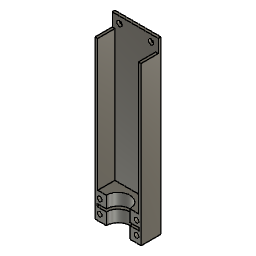
platform_bottom (Autodesk Fusion 360 design; units mm, degrees)
Autodesk Fusion 360 part; units mm, degrees
sketch "スケッチ1" plane through (0, 0, 0) normal (0, 0, 1) x (1, 0, 0)
  line L0 (-17.5, 15) -> (17.5, 15)
  line L1 (17.5, 15) -> (17.5, 0)
  line L2 (17.5, 0) -> (-17.5, 0)
  line L3 (-17.5, 0) -> (-17.5, 15)
  dimension "d1" = 35
  dimension "d2" = 15
  constraint horizontal L0
  constraint vertical L1
  constraint horizontal L2
  constraint vertical L3
  constraint midpoint origin L2
  measures "d1" distance of L0.start L0.end
  measures "d2" distance of L0.start L2.end
extrude "押し出し1" add sketch "スケッチ1" along normal blind 120
sketch "スケッチ2" plane through (0, 0, 0) normal (0, 0, -1) x (1, 0, 0)
  line L0 (17.5, 0) -> (-17.5, 0)
  line L1 (-17.5, 0) -> (-17.5, -15)
  line L2 (-17.5, -15) -> (17.5, -15)
  line L3 (17.5, -15) -> (17.5, 0)
  circle A0 centre (0, 0) radius 9
  dimension "d5" = 18
  constraint coincident A0.centre origin
  measures "d5" diameter of A0
extrude "押し出し2" cut sketch "スケッチ2" against normal blind 20 contours L0 A0 picked at (1.5, -2.5981)
sketch "スケッチ3" plane through (0, 0, 120) normal (0, 0, 1) x (-1, 0, 0)
  line L0 (17.5, 0) -> (-17.5, 0)
  line L1 (-17.5, 0) -> (-17.5, -15)
  line L2 (-17.5, -15) -> (17.5, -15)
  line L3 (17.5, -15) -> (17.5, 0)
  line L4 (15.5, -13) -> (-15.5, -13)
  line L5 (-15.5, -13) -> (-15.5, 0)
  line L6 (-15.5, 0) -> (15.5, 0)
  line L7 (15.5, 0) -> (15.5, -13)
  dimension "d8" = 2
  dimension "d9" = 31
  constraint horizontal L4
  constraint vertical L5
  constraint horizontal L6
  constraint vertical L7
  constraint coincident L0 L5.end
  constraint midpoint origin L6
  measures "d8" distance of L2 L4
  measures "d9" distance of L5 L7
extrude "押し出し3" cut sketch "スケッチ3" against normal blind 100 contours L0 L4 L5 L6 L7
ref_plane "作業平面1" through (0, 7.5, 9) normal (0, 0, -1) x (-1, 0, 0)
sketch "スケッチ4" plane through (0, 6, 9) normal (0, 0, -1) x (1, 0, 0)
  line L0 (-17.5, 6) -> (17.5, 6)
  line L1 (17.5, 6) -> (17.5, -5)
  line L2 (17.5, -5) -> (-17.5, -5)
  line L3 (-17.5, -5) -> (-17.5, 6)
  line L4 (-17.5, 6) -> (-17.5, -9)
  line L5 (17.5, -9) -> (17.5, 6)
  line L6 (17.5, 6) -> (9, 6)
  dimension "d13" = 11
  constraint horizontal L0
  constraint vertical L1
  constraint horizontal L2
  constraint vertical L3
  constraint collinear L3 L4
  constraint collinear L1 L5
  constraint collinear L0 L6
  measures "d13" distance of L0 L2
extrude "押し出し4" cut sketch "スケッチ4" against normal blind 2
sketch "スケッチ5" plane through (0, 15, 0) normal (0, 1, 0) x (-1, 0, 0)
  line L0 (-17.5, 0) -> (17.5, 0)
  line L1 (17.5, 0) -> (17.5, 120)
  line L2 (17.5, 120) -> (-17.5, 120)
  line L3 (-17.5, 120) -> (-17.5, 0)
  line L4 (-17.5, 130) -> (17.5, 130)
  line L5 (17.5, 130) -> (17.5, 120)
  line L6 (17.5, 120) -> (-17.5, 120)
  line L7 (-17.5, 120) -> (-17.5, 130)
  line L8 (-17.5, 125) -> (17.5, 125) construction
  circle A0 centre (12, 125) radius 2
  circle A1 centre (-12, 125) radius 2
  dimension "d16" = 4
  dimension "d17" = 4
  dimension "d18" = 24
  dimension "d19" = 10
  dimension "d20" = 5.5
  constraint horizontal L4
  constraint vertical L5
  constraint horizontal L6
  constraint vertical L7
  constraint collinear L2 L6
  constraint midpoint L7 L8.start
  constraint midpoint L5 L8.end
  constraint coincident L8 A0.centre
  constraint coincident L8 A1.centre
  constraint collinear L3 L7
  constraint collinear L1 L5
  measures "d16" diameter of A1
  measures "d17" diameter of A0
  measures "d18" distance of A0.centre A1.centre
  measures "d19" distance of L4.start L2.end
  measures "d20" distance of L8.end A0.centre
extrude "押し出し5" add sketch "スケッチ5" against normal blind 2 contours L2 L4 L5 L6 L7
sketch "スケッチ7" plane through (0, 0, 0) normal (0, -1, 0) x (1, 0, 0)
  line L0 (-17.5, 11) -> (-9, 11)
  line L1 (-9, 11) -> (-9, 20)
  line L2 (-9, 20) -> (-15.5, 20)
  line L3 (-15.5, 20) -> (-15.5, 120)
  line L4 (-15.5, 120) -> (-17.5, 120)
  line L5 (-17.5, 120) -> (-17.5, 11)
  line L6 (-17.5, 11) -> (-16, 11)
  line L7 (-16, 11) -> (-16, 9)
  line L8 (-16, 9) -> (-17.5, 9)
  line L9 (-17.5, 9) -> (-17.5, 11)
  line L10 (-9, 9) -> (-17.5, 9)
  line L11 (17.5, 11) -> (16, 11)
  line L12 (16, 11) -> (16, 9)
  line L13 (16, 9) -> (17.5, 9)
  line L14 (17.5, 9) -> (17.5, 11)
  line L15 (17.5, 9) -> (9, 9)
  point P0 (17.5, 11)
  dimension "d26" = 32
  dimension "d27" = 1.5
  constraint horizontal L6
  constraint vertical L7
  constraint horizontal L8
  constraint vertical L9
  constraint coincident L0.start L5.end
  constraint collinear L8 L10
  constraint horizontal L11
  constraint vertical L12
  constraint horizontal L13
  constraint vertical L14
  constraint coincident P0 L11.start
  constraint collinear L13 L15
  measures "d26" distance of L7 L12
  measures "d27" distance of L12 L14
extrude "押し出し7" add sketch "スケッチ7" against normal blind 11 contours L0 L6 L7 L8 L9 L10 | L11 L12 L13 L14 L15
sketch "スケッチ8" plane through (0, 0, 0) normal (0, -1, 0) x (1, 0, 0)
  line L0 (-16, 11) -> (-9, 11)
  line L1 (-9, 11) -> (-9, 20)
  line L2 (-9, 20) -> (-15.5, 20)
  line L3 (-15.5, 20) -> (-15.5, 120)
  line L4 (-15.5, 120) -> (-17.5, 120)
  line L5 (-17.5, 120) -> (-17.5, 0)
  line L6 (-17.5, 0) -> (-9, 0)
  line L7 (-9, 0) -> (-9, 9)
  line L8 (-9, 9) -> (-16, 9)
  line L9 (-16, 9) -> (-16, 11)
  circle A0 centre (-14, 15) radius 1.75
  line L10 (18.5, 15) -> (-17.5, 15) construction
  line L11 (17.541, 5) -> (-17.5, 5) construction
  line L12 (15.5, 20) -> (9, 20) construction
  circle A1 centre (14, 15) radius 1.75
  circle A2 centre (14, 5) radius 1.75
  circle A3 centre (-14, 5) radius 1.75
  line L13 (17.5, 0) -> (17.5, 120)
  dimension "d30" = 5
  dimension "d31" = 10
  dimension "d32" = 3.5
  dimension "d33" = 3.5
  dimension "d34" = 3.5
  dimension "d35" = 3.5
  dimension "d36" = 3.5
  dimension "d37" = 3.5
  dimension "d38" = 3.5
  dimension "d39" = 3.5
  constraint coincident L5 L10.end
  constraint perpendicular L5 L10
  constraint coincident L5 L11.end
  constraint perpendicular L5 L11
  constraint coincident L10 A1.centre
  constraint coincident L11 A2.centre
  constraint coincident L11 A3.centre
  constraint coincident A0.centre L10
  measures "d30" distance of L10 L12
  measures "d31" distance of L10 L11
  measures "d32" diameter of A0
  measures "d33" diameter of A1
  measures "d34" diameter of A2
  measures "d35" diameter of A3
  measures "d36" distance of A0.centre L10.end
  measures "d37" distance of L5 A3.centre
  measures "d38" distance of A1.centre L13
  measures "d39" distance of A2.centre L13
extrude "押し出し8" cut sketch "スケッチ8" against normal blind 15 contours A0 | A1 | A2 | A3
